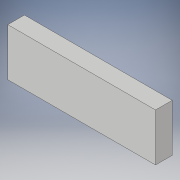
# Autodesk Inventor part: Convex Organ Bank Castor Slots
Saved by Autodesk Inventor 2019 (Build 230136000, 136)
## iProperties
Created: 2021-02-18
Part Number: Convex Organ Bank Castor Slots
Material: Generic
Document SubType Name: Modeling
Designer: Eric
Density: 1 g/cm^3
Appearance: Default
Author: Eric
Autodesk Inventor part; units mm, degrees
ref_plane "YZ Plane" through (0, 0, 0) normal (1, 0, 0) x (0, 1, 0)
ref_plane "XZ Plane" through (0, 0, 0) normal (0, 1, 0) x (-1, 0, 0)
ref_plane "XY Plane" through (0, 0, 0) normal (0, 0, 1) x (1, 0, 0)
sketch "Sketch1" plane through (0, 0, 0) normal (0, 0, 1) x (1, 0, 0)
  line L0 (0, -5) -> (124, -5) construction
  line L1 (124, -5) -> (124, -40) construction
  line L2 (124, -40) -> (0, -40) construction
  line L3 (0, -40) -> (0, -5) construction
  line L4 (0, 0) -> (124, 0)
  line L5 (124, 0) -> (124, -40)
  line L6 (124, -40) -> (0, -40)
  line L7 (0, -40) -> (0, 0)
  dimension "d0" = 124
  dimension "d1" = 35
  dimension "d2" = 5
  constraints: 16 end point, 4 horizontal, 4 vertical, 3 collinear
  measures "d0" distance of L1.end L2.end
  measures "d1" distance of L0.end L1.end
  measures "d2" distance between parallel lines of L4 L0
extrude "Extrusion1" add sketch "Sketch1" along normal blind 14
body "Solid1"
